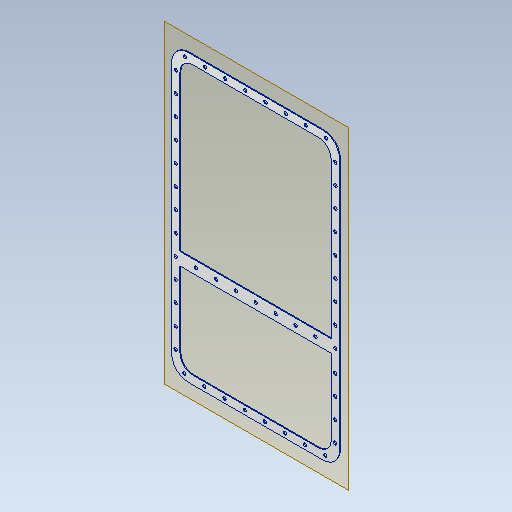
# Autodesk Inventor part: Прокладка крышки фонаря 2_CPY
Saved by Autodesk Inventor 2021 (Build 250183000, 183)
## iProperties
Created: 2020-12-10
Part Number: Прокладка крышки фонаря 2_CPY
Material: Алюминий 6061
Document SubType Name: Modeling
Designer: Тимоха
Mass: 266.415 g
Surface Area: 1105.35 cm^2
Volume: 98.6722 cm^3
Density: 2.7 g/cm^3
Appearance: Алюминий — плоский
Author: Тимоха
Autodesk Inventor part; units mm, degrees
ref_plane "YZ Plane" through (0, 0, 0) normal (1, 0, 0) x (0, 1, 0)
ref_plane "XZ Plane" through (0, 0, 0) normal (0, 1, 0) x (-1, 0, 0)
ref_plane "XY Plane" through (0, 0, 0) normal (0, 0, 1) x (1, 0, 0)
ref_plane "РабПлоскость1" through (0, 0, 0) normal (0, 0, 1) x (1, 0, 0)
sketch "Эскиз1" plane through (0, 0, 0) normal (0, 0, 1) x (1, 0, 0)
  circle A0 centre (-141.8, -95) radius 4 projected
  circle A1 centre (-94.4, -95) radius 4 projected
  circle A2 centre (-47, -95) radius 4 projected
  circle A3 centre (0.4, -95) radius 4 projected
  circle A4 centre (47.8, -95) radius 4 projected
  circle A5 centre (95.2, -95) radius 4 projected
  circle A6 centre (142.6, -95) radius 4 projected
  circle A7 centre (189.4425, -146.4995) radius 4 projected
  circle A8 centre (189.4425, -194.4995) radius 4 projected
  circle A9 centre (189.4425, -242.4995) radius 4 projected
  circle A10 centre (189.4425, -290.4995) radius 4 projected
  circle A11 centre (165.7163, -328.1346) radius 4 projected
  circle A12 centre (117.9209, -330) radius 4 projected
  circle A13 centre (69.9209, -330) radius 4 projected
  circle A14 centre (21.9209, -330) radius 4 projected
  circle A15 centre (-26.0791, -330) radius 4 projected
  circle A16 centre (-74.0791, -330) radius 4 projected
  circle A17 centre (-122.0791, -330) radius 4 projected
  circle A18 centre (-169.6605, -327.0042) radius 4 projected
  circle A19 centre (-190.486, -287.3914) radius 4 projected
  circle A20 centre (-190.4444, -239.3914) radius 4 projected
  circle A21 centre (-190.4029, -191.3914) radius 4 projected
  circle A22 centre (-190.3613, -143.3914) radius 4 projected
  circle A23 centre (-190.3198, -95.3914) radius 4 projected
  circle A24 centre (-190.2782, -47.3914) radius 4 projected
  circle A25 centre (-190.2367, 0.6085) radius 4 projected
  circle A26 centre (-190.1952, 48.6085) radius 4 projected
  circle A27 centre (-190.1536, 96.6085) radius 4 projected
  circle A28 centre (-190.1121, 144.6085) radius 4 projected
  circle A29 centre (-190.0705, 192.6085) radius 4 projected
  circle A30 centre (-190.029, 240.6084) radius 4 projected
  circle A31 centre (-189.9874, 288.6084) radius 4 projected
  circle A32 centre (-168.0002, 327.4583) radius 4 projected
  circle A33 centre (-120.3208, 329.9395) radius 4 projected
  circle A34 centre (-72.3208, 329.8979) radius 4 projected
  circle A35 centre (-24.3209, 329.8564) radius 4 projected
  circle A36 centre (23.6791, 329.8148) radius 4 projected
  circle A37 centre (71.6791, 329.7733) radius 4 projected
  circle A38 centre (119.6791, 329.7317) radius 4 projected
  circle A39 centre (167.4036, 327.4296) radius 4 projected
  circle A40 centre (190, 289) radius 4 projected
  circle A41 centre (190, 241) radius 4 projected
  circle A42 centre (190, 193) radius 4 projected
  circle A43 centre (190, 145) radius 4 projected
  circle A44 centre (190, 97) radius 4 projected
  circle A45 centre (190, 49) radius 4 projected
  circle A46 centre (190, 1) radius 4 projected
  circle A47 centre (190, -47) radius 4 projected
  circle A48 centre (190, -95) radius 4 projected
  line L0 (200, 300) -> (200, -300) projected
  arc A49 (200, 300) -> (160, 340) centre (160, 300) ccw projected
  line L1 (-160, 340) -> (160, 340) projected
  arc A50 (-160, 340) -> (-200, 300) centre (-160, 300) ccw projected
  line L2 (-200, -300) -> (-200, 300) projected
  arc A51 (-200, -300) -> (-160, -340) centre (-160, -300) ccw projected
  line L3 (160, -340) -> (-160, -340) projected
  arc A52 (160, -340) -> (200, -300) centre (160, -300) ccw projected
  line L4 (180, -110) -> (-180, -110) projected
  line L5 (180, -290) -> (180, -110) projected
  arc A53 (150, -320) -> (180, -290) centre (150, -290) ccw projected
  line L6 (-150, -320) -> (150, -320) projected
  arc A54 (-180, -290) -> (-150, -320) centre (-150, -290) ccw projected
  line L7 (-180, -110) -> (-180, -290) projected
  line L8 (180, -80) -> (180, 290) projected
  line L9 (-180, -80) -> (180, -80) projected
  line L10 (-180, 290) -> (-180, -80) projected
  arc A55 (-150, 320) -> (-180, 290) centre (-150, 290) ccw projected
  line L11 (150, 320) -> (-150, 320) projected
  arc A56 (180, 290) -> (150, 320) centre (150, 290) ccw projected
  point P0 (0, 0)
extrude "Выдавливание1" add sketch "Эскиз1" along normal blind 2
